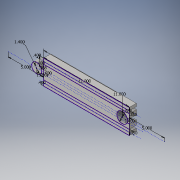
# Autodesk Inventor part: Sun_StraightTrack
Saved by Autodesk Inventor 2016 (Build 200138000, 138)
## iProperties
Created: 2018-01-17
Part Number: Sun_StraightTrack
Material: Generic
Document SubType Name: Modeling
Designer: sun01147
Density: 1 g/cm^3
Appearance: Default
Author: sun01147
Autodesk Inventor part; units mm, degrees
ref_plane "YZ Plane" through (0, 0, 0) normal (1, 0, 0) x (0, 1, 0)
ref_plane "XZ Plane" through (0, 0, 0) normal (0, 1, 0) x (-1, 0, 0)
ref_plane "XY Plane" through (0, 0, 0) normal (0, 0, 1) x (1, 0, 0)
sketch "Sketch1" plane through (0, 0, 0) normal (0, 0, 1) x (1, 0, 0)
  line L0 (0, 0) -> (304.8, 0)
  line L1 (304.8, 0) -> (304.8, 86.36)
  line L2 (304.8, 86.36) -> (0, 86.36)
  line L3 (0, 86.36) -> (0, 0)
  line L4 (0, 43.18) -> (304.8, 43.18) construction
  line L5 (0, 43.18) -> (-127, 43.18) construction
  line L6 (304.8, 43.18) -> (431.8, 43.18) construction
  line L7 (-35.3212, 50.8) -> (355.1298, 50.8) construction
  line L8 (-9.3356, 35.56) -> (354.8509, 35.56) construction
  circle A0 centre (-25.4, 43.18) radius 17.78
  line L9 (-9.3356, 50.8) -> (0, 50.8)
  line L10 (-9.3356, 35.56) -> (0, 35.56)
  line L11 (-16.6442, 10.16) -> (350.0615, 10.16) construction
  line L12 (-16.6442, 76.2) -> (344.385, 76.2) construction
  line L13 (0, 10.16) -> (304.8, 10.16)
  line L14 (0, 76.2) -> (304.8, 76.2)
  line L15 (0, 67.31) -> (304.8, 67.31)
  line L16 (0, 19.05) -> (304.8, 19.05)
  line L17 (304.8, 50.8) -> (296.8596, 50.8)
  line L18 (304.8, 35.56) -> (296.8596, 35.56)
  circle A1 centre (279.4, 43.18) radius 19.05
  dimension "d0" = 304.8
  dimension "d1" = 86.36
  dimension "d2" = 127
  dimension "d3" = 127
  dimension "d5" = 35.56
  dimension "d6" = 15.24
  dimension "d7" = 35.56
  dimension "d8" = 25.4
  dimension "d9" = 9.3356
  dimension "d10" = 10.16
  dimension "d11" = 10.16
  dimension "d12" = 8.89
  dimension "d13" = 8.89
  dimension "d22" = 38.1
  dimension "d23" = 279.4
  constraints: 34 end point, 12 horizontal, 10 point on line, 4 point on circle, 2 centre point, 1 parallel, 20 other
  measures "d0" distance of L2.start L2.end
  measures "d1" distance of L0.end L2.start
  measures "d2" distance of L4.start L5.end
  measures "d3" distance of L4.end L6.end
  measures "d5" diameter of A0
  measures "d6" distance between parallel lines of L8 L7
  measures "d7" distance from line of L7 L2.end
  measures "d8" distance of L4.start A0.centre
  measures "d9" distance of L9.start L9.end
  measures "d10" distance between parallel lines of L11 L0
  measures "d11" distance between parallel lines of L12 L2
  measures "d12" distance between parallel lines of L15 L14
  measures "d13" distance between parallel lines of L13 L16
  measures "d22" diameter of A1
extrude "Extrusion1" add sketch "Sketch1" against normal blind 25.4 contours L3 L13 L1 L0 | L3 L15 L1 L17 A1 L18 L16 | L10 A0 L9 L3 | A0 | L3 L2 L1 L14
extrude "Extrusion2" add sketch "Sketch1" against normal blind 4.7625 contours L3 L16 L1 L13 | L3 L14 L1 L15
body "Solid1"
